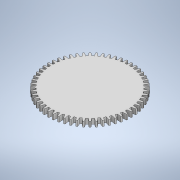
# Autodesk Inventor part: bánh răng 2
Saved by Autodesk Inventor 2020 (Build 240168000, 168)
## iProperties
Created: 2022-11-27
Part Number: bánh răng 2
Material: Generic
Document SubType Name: Modeling
Designer: ADMIN
Density: 1 g/cm^3
Appearance: Default
Author: ADMIN
Autodesk Inventor part; units mm, degrees
ref_plane "YZ Plane" through (0, 0, 0) normal (1, 0, 0) x (0, 1, 0)
ref_plane "XZ Plane" through (0, 0, 0) normal (0, 1, 0) x (-1, 0, 0)
ref_plane "XY Plane" through (0, 0, 0) normal (0, 0, 1) x (1, 0, 0)
sketch "Sketch1" plane through (0, 0, 0) normal (0, 1, 0) x (-1, 0, 0)
  arc A0 (32.9962, -0.5) -> (32.9962, 0.5) centre (0, 0) ccw
  line L0 (29.9833, 1) -> (32.9962, 0.5)
  line L1 (29.9833, -1) -> (32.9962, -0.5)
  line L2 (29.6828, -4.3508) -> (32.7328, -4.1913)
  line L3 (29.9068, -2.3634) -> (32.8447, -3.1975)
  arc A1 (32.7328, -4.1913) -> (32.8447, -3.1975) centre (0, 0) ccw
  line L4 (29.0091, -7.6468) -> (32.0577, -7.8298)
  line L5 (29.4541, -5.697) -> (32.2802, -6.8549)
  arc A2 (32.0577, -7.8298) -> (32.2802, -6.8549) centre (0, 0) ccw
  line L6 (27.9705, -10.8467) -> (30.9794, -11.3699)
  line L7 (28.631, -8.959) -> (31.3097, -10.426)
  arc A3 (30.9794, -11.3699) -> (31.3097, -10.426) centre (0, 0) ccw
  line L8 (26.5802, -13.9102) -> (29.5116, -14.767)
  line L9 (27.4479, -12.1083) -> (29.9455, -13.866)
  arc A4 (29.5116, -14.767) -> (29.9455, -13.866) centre (0, 0) ccw
  line L10 (24.8556, -16.7988) -> (27.6727, -17.9784)
  line L11 (25.9196, -15.1054) -> (28.2047, -17.1317)
  arc A5 (27.6727, -17.9784) -> (28.2047, -17.1317) centre (0, 0) ccw
  line L12 (22.8184, -19.4761) -> (25.4857, -20.9637)
  line L13 (24.0654, -17.9125) -> (26.1092, -20.1819)
  arc A6 (25.4857, -20.9637) -> (26.1092, -20.1819) centre (0, 0) ccw
  line L14 (20.4943, -21.9085) -> (22.9783, -23.6854)
  line L15 (21.9085, -20.4943) -> (23.6854, -22.9783)
  arc A7 (22.9783, -23.6854) -> (23.6854, -22.9783) centre (0, 0) ccw
  line L16 (17.9125, -24.0654) -> (20.1819, -26.1092)
  line L17 (19.4761, -22.8184) -> (20.9637, -25.4857)
  arc A8 (20.1819, -26.1092) -> (20.9637, -25.4857) centre (0, 0) ccw
  line L18 (15.1054, -25.9196) -> (17.1317, -28.2047)
  line L19 (16.7988, -24.8556) -> (17.9784, -27.6727)
  arc A9 (17.1317, -28.2047) -> (17.9784, -27.6727) centre (0, 0) ccw
  line L20 (12.1083, -27.4479) -> (13.866, -29.9455)
  line L21 (13.9102, -26.5802) -> (14.767, -29.5116)
  arc A10 (13.866, -29.9455) -> (14.767, -29.5116) centre (0, 0) ccw
  line L22 (8.959, -28.631) -> (10.426, -31.3097)
  line L23 (10.8467, -27.9705) -> (11.3699, -30.9794)
  arc A11 (10.426, -31.3097) -> (11.3699, -30.9794) centre (0, 0) ccw
  line L24 (5.697, -29.4541) -> (6.8549, -32.2802)
  line L25 (7.6468, -29.0091) -> (7.8298, -32.0577)
  arc A12 (6.8549, -32.2802) -> (7.8298, -32.0577) centre (0, 0) ccw
  line L26 (2.3634, -29.9068) -> (3.1975, -32.8447)
  line L27 (4.3508, -29.6828) -> (4.1913, -32.7328)
  arc A13 (3.1975, -32.8447) -> (4.1913, -32.7328) centre (0, 0) ccw
  line L28 (-1, -29.9833) -> (-0.5, -32.9962)
  line L29 (1, -29.9833) -> (0.5, -32.9962)
  arc A14 (-0.5, -32.9962) -> (0.5, -32.9962) centre (0, 0) ccw
  line L30 (-4.3508, -29.6828) -> (-4.1913, -32.7328)
  line L31 (-2.3634, -29.9068) -> (-3.1975, -32.8447)
  arc A15 (-4.1913, -32.7328) -> (-3.1975, -32.8447) centre (0, 0) ccw
  line L32 (-7.6468, -29.0091) -> (-7.8298, -32.0577)
  line L33 (-5.697, -29.4541) -> (-6.8549, -32.2802)
  arc A16 (-7.8298, -32.0577) -> (-6.8549, -32.2802) centre (0, 0) ccw
  line L34 (-10.8467, -27.9705) -> (-11.3699, -30.9794)
  line L35 (-8.959, -28.631) -> (-10.426, -31.3097)
  arc A17 (-11.3699, -30.9794) -> (-10.426, -31.3097) centre (0, 0) ccw
  line L36 (-13.9102, -26.5802) -> (-14.767, -29.5116)
  line L37 (-12.1083, -27.4479) -> (-13.866, -29.9455)
  arc A18 (-14.767, -29.5116) -> (-13.866, -29.9455) centre (0, 0) ccw
  line L38 (-16.7988, -24.8556) -> (-17.9784, -27.6727)
  line L39 (-15.1054, -25.9196) -> (-17.1317, -28.2047)
  arc A19 (-17.9784, -27.6727) -> (-17.1317, -28.2047) centre (0, 0) ccw
  line L40 (-19.4761, -22.8184) -> (-20.9637, -25.4857)
  line L41 (-17.9125, -24.0654) -> (-20.1819, -26.1092)
  arc A20 (-20.9637, -25.4857) -> (-20.1819, -26.1092) centre (0, 0) ccw
  line L42 (-21.9085, -20.4943) -> (-23.6854, -22.9783)
  line L43 (-20.4943, -21.9085) -> (-22.9783, -23.6854)
  arc A21 (-23.6854, -22.9783) -> (-22.9783, -23.6854) centre (0, 0) ccw
  line L44 (-24.0654, -17.9125) -> (-26.1092, -20.1819)
  line L45 (-22.8184, -19.4761) -> (-25.4857, -20.9637)
  arc A22 (-26.1092, -20.1819) -> (-25.4857, -20.9637) centre (0, 0) ccw
  line L46 (-25.9196, -15.1054) -> (-28.2047, -17.1317)
  line L47 (-24.8556, -16.7988) -> (-27.6727, -17.9784)
  arc A23 (-28.2047, -17.1317) -> (-27.6727, -17.9784) centre (0, 0) ccw
  line L48 (-27.4479, -12.1083) -> (-29.9455, -13.866)
  line L49 (-26.5802, -13.9102) -> (-29.5116, -14.767)
  arc A24 (-29.9455, -13.866) -> (-29.5116, -14.767) centre (0, 0) ccw
  line L50 (-28.631, -8.959) -> (-31.3097, -10.426)
  line L51 (-27.9705, -10.8467) -> (-30.9794, -11.3699)
  arc A25 (-31.3097, -10.426) -> (-30.9794, -11.3699) centre (0, 0) ccw
  line L52 (-29.4541, -5.697) -> (-32.2802, -6.8549)
  line L53 (-29.0091, -7.6468) -> (-32.0577, -7.8298)
  arc A26 (-32.2802, -6.8549) -> (-32.0577, -7.8298) centre (0, 0) ccw
  line L54 (-29.9068, -2.3634) -> (-32.8447, -3.1975)
  line L55 (-29.6828, -4.3508) -> (-32.7328, -4.1913)
  arc A27 (-32.8447, -3.1975) -> (-32.7328, -4.1913) centre (0, 0) ccw
  line L56 (-29.9833, 1) -> (-32.9962, 0.5)
  line L57 (-29.9833, -1) -> (-32.9962, -0.5)
  arc A28 (-32.9962, 0.5) -> (-32.9962, -0.5) centre (0, 0) ccw
  line L58 (-29.6828, 4.3508) -> (-32.7328, 4.1913)
  line L59 (-29.9068, 2.3634) -> (-32.8447, 3.1975)
  arc A29 (-32.7328, 4.1913) -> (-32.8447, 3.1975) centre (0, 0) ccw
  line L60 (-29.0091, 7.6468) -> (-32.0577, 7.8298)
  line L61 (-29.4541, 5.697) -> (-32.2802, 6.8549)
  arc A30 (-32.0577, 7.8298) -> (-32.2802, 6.8549) centre (0, 0) ccw
  line L62 (-27.9705, 10.8467) -> (-30.9794, 11.3699)
  line L63 (-28.631, 8.959) -> (-31.3097, 10.426)
  arc A31 (-30.9794, 11.3699) -> (-31.3097, 10.426) centre (0, 0) ccw
  line L64 (-26.5802, 13.9102) -> (-29.5116, 14.767)
  line L65 (-27.4479, 12.1083) -> (-29.9455, 13.866)
  arc A32 (-29.5116, 14.767) -> (-29.9455, 13.866) centre (0, 0) ccw
  line L66 (-24.8556, 16.7988) -> (-27.6727, 17.9784)
  line L67 (-25.9196, 15.1054) -> (-28.2047, 17.1317)
  arc A33 (-27.6727, 17.9784) -> (-28.2047, 17.1317) centre (0, 0) ccw
  line L68 (-22.8184, 19.4761) -> (-25.4857, 20.9637)
  line L69 (-24.0654, 17.9125) -> (-26.1092, 20.1819)
  arc A34 (-25.4857, 20.9637) -> (-26.1092, 20.1819) centre (0, 0) ccw
  line L70 (-20.4943, 21.9085) -> (-22.9783, 23.6854)
  line L71 (-21.9085, 20.4943) -> (-23.6854, 22.9783)
  arc A35 (-22.9783, 23.6854) -> (-23.6854, 22.9783) centre (0, 0) ccw
  line L72 (-17.9125, 24.0654) -> (-20.1819, 26.1092)
  line L73 (-19.4761, 22.8184) -> (-20.9637, 25.4857)
  arc A36 (-20.1819, 26.1092) -> (-20.9637, 25.4857) centre (0, 0) ccw
  line L74 (-15.1054, 25.9196) -> (-17.1317, 28.2047)
  line L75 (-16.7988, 24.8556) -> (-17.9784, 27.6727)
  arc A37 (-17.1317, 28.2047) -> (-17.9784, 27.6727) centre (0, 0) ccw
  line L76 (-12.1083, 27.4479) -> (-13.866, 29.9455)
  line L77 (-13.9102, 26.5802) -> (-14.767, 29.5116)
  arc A38 (-13.866, 29.9455) -> (-14.767, 29.5116) centre (0, 0) ccw
  line L78 (-8.959, 28.631) -> (-10.426, 31.3097)
  line L79 (-10.8467, 27.9705) -> (-11.3699, 30.9794)
  arc A39 (-10.426, 31.3097) -> (-11.3699, 30.9794) centre (0, 0) ccw
  line L80 (-5.697, 29.4541) -> (-6.8549, 32.2802)
  line L81 (-7.6468, 29.0091) -> (-7.8298, 32.0577)
  arc A40 (-6.8549, 32.2802) -> (-7.8298, 32.0577) centre (0, 0) ccw
  line L82 (-2.3634, 29.9068) -> (-3.1975, 32.8447)
  line L83 (-4.3508, 29.6828) -> (-4.1913, 32.7328)
  arc A41 (-3.1975, 32.8447) -> (-4.1913, 32.7328) centre (0, 0) ccw
  line L84 (1, 29.9833) -> (0.5, 32.9962)
  line L85 (-1, 29.9833) -> (-0.5, 32.9962)
  arc A42 (0.5, 32.9962) -> (-0.5, 32.9962) centre (0, 0) ccw
  line L86 (4.3508, 29.6828) -> (4.1913, 32.7328)
  line L87 (2.3634, 29.9068) -> (3.1975, 32.8447)
  arc A43 (4.1913, 32.7328) -> (3.1975, 32.8447) centre (0, 0) ccw
  line L88 (7.6468, 29.0091) -> (7.8298, 32.0577)
  line L89 (5.697, 29.4541) -> (6.8549, 32.2802)
  arc A44 (7.8298, 32.0577) -> (6.8549, 32.2802) centre (0, 0) ccw
  line L90 (10.8467, 27.9705) -> (11.3699, 30.9794)
  line L91 (8.959, 28.631) -> (10.426, 31.3097)
  arc A45 (11.3699, 30.9794) -> (10.426, 31.3097) centre (0, 0) ccw
  line L92 (13.9102, 26.5802) -> (14.767, 29.5116)
  line L93 (12.1083, 27.4479) -> (13.866, 29.9455)
  arc A46 (14.767, 29.5116) -> (13.866, 29.9455) centre (0, 0) ccw
  line L94 (16.7988, 24.8556) -> (17.9784, 27.6727)
  line L95 (15.1054, 25.9196) -> (17.1317, 28.2047)
  arc A47 (17.9784, 27.6727) -> (17.1317, 28.2047) centre (0, 0) ccw
  line L96 (19.4761, 22.8184) -> (20.9637, 25.4857)
  line L97 (17.9125, 24.0654) -> (20.1819, 26.1092)
  arc A48 (20.9637, 25.4857) -> (20.1819, 26.1092) centre (0, 0) ccw
  line L98 (21.9085, 20.4943) -> (23.6854, 22.9783)
  line L99 (20.4943, 21.9085) -> (22.9783, 23.6854)
  arc A49 (23.6854, 22.9783) -> (22.9783, 23.6854) centre (0, 0) ccw
  line L100 (24.0654, 17.9125) -> (26.1092, 20.1819)
  line L101 (22.8184, 19.4761) -> (25.4857, 20.9637)
  arc A50 (26.1092, 20.1819) -> (25.4857, 20.9637) centre (0, 0) ccw
  line L102 (25.9196, 15.1054) -> (28.2047, 17.1317)
  line L103 (24.8556, 16.7988) -> (27.6727, 17.9784)
  arc A51 (28.2047, 17.1317) -> (27.6727, 17.9784) centre (0, 0) ccw
  line L104 (27.4479, 12.1083) -> (29.9455, 13.866)
  line L105 (26.5802, 13.9102) -> (29.5116, 14.767)
  arc A52 (29.9455, 13.866) -> (29.5116, 14.767) centre (0, 0) ccw
  line L106 (28.631, 8.959) -> (31.3097, 10.426)
  line L107 (27.9705, 10.8467) -> (30.9794, 11.3699)
  arc A53 (31.3097, 10.426) -> (30.9794, 11.3699) centre (0, 0) ccw
  line L108 (29.4541, 5.697) -> (32.2802, 6.8549)
  line L109 (29.0091, 7.6468) -> (32.0577, 7.8298)
  arc A54 (32.2802, 6.8549) -> (32.0577, 7.8298) centre (0, 0) ccw
  line L110 (29.9068, 2.3634) -> (32.8447, 3.1975)
  line L111 (29.6828, 4.3508) -> (32.7328, 4.1913)
  arc A55 (32.8447, 3.1975) -> (32.7328, 4.1913) centre (0, 0) ccw
  arc A56 (22.8184, 19.4761) -> (21.9085, 20.4943) centre (0, 0) ccw
  arc A57 (20.4943, 21.9085) -> (19.4761, 22.8184) centre (0, 0) ccw
  arc A58 (17.9125, 24.0654) -> (16.7988, 24.8556) centre (0, 0) ccw
  arc A59 (15.1054, 25.9196) -> (13.9102, 26.5802) centre (0, 0) ccw
  arc A60 (12.1083, 27.4479) -> (10.8467, 27.9705) centre (0, 0) ccw
  arc A61 (8.959, 28.631) -> (7.6468, 29.0091) centre (0, 0) ccw
  arc A62 (5.697, 29.4541) -> (4.3508, 29.6828) centre (0, 0) ccw
  arc A63 (2.3634, 29.9068) -> (1, 29.9833) centre (0, 0) ccw
  arc A64 (-1, 29.9833) -> (-2.3634, 29.9068) centre (0, 0) ccw
  arc A65 (-4.3508, 29.6828) -> (-5.697, 29.4541) centre (0, 0) ccw
  arc A66 (-7.6468, 29.0091) -> (-8.959, 28.631) centre (0, 0) ccw
  arc A67 (-10.8467, 27.9705) -> (-12.1083, 27.4479) centre (0, 0) ccw
  arc A68 (-13.9102, 26.5802) -> (-15.1054, 25.9196) centre (0, 0) ccw
  arc A69 (-16.7988, 24.8556) -> (-17.9125, 24.0654) centre (0, 0) ccw
  arc A70 (-19.4761, 22.8184) -> (-20.4943, 21.9085) centre (0, 0) ccw
  arc A71 (-21.9085, 20.4943) -> (-22.8184, 19.4761) centre (0, 0) ccw
  arc A72 (-24.0654, 17.9125) -> (-24.8556, 16.7988) centre (0, 0) ccw
  arc A73 (-25.9196, 15.1054) -> (-26.5802, 13.9102) centre (0, 0) ccw
  arc A74 (-27.4479, 12.1083) -> (-27.9705, 10.8467) centre (0, 0) ccw
  arc A75 (-28.631, 8.959) -> (-29.0091, 7.6468) centre (0, 0) ccw
  arc A76 (-29.4541, 5.697) -> (-29.6828, 4.3508) centre (0, 0) ccw
  arc A77 (-29.9068, 2.3634) -> (-29.9833, 1) centre (0, 0) ccw
  arc A78 (-29.9833, -1) -> (-29.9068, -2.3634) centre (0, 0) ccw
  arc A79 (-29.6828, -4.3508) -> (-29.4541, -5.697) centre (0, 0) ccw
  arc A80 (-29.0091, -7.6468) -> (-28.631, -8.959) centre (0, 0) ccw
  arc A81 (-27.9705, -10.8467) -> (-27.4479, -12.1083) centre (0, 0) ccw
  arc A82 (-26.5802, -13.9102) -> (-25.9196, -15.1054) centre (0, 0) ccw
  arc A83 (-24.8556, -16.7988) -> (-24.0654, -17.9125) centre (0, 0) ccw
  arc A84 (-22.8184, -19.4761) -> (-21.9085, -20.4943) centre (0, 0) ccw
  arc A85 (-20.4943, -21.9085) -> (-19.4761, -22.8184) centre (0, 0) ccw
  arc A86 (-17.9125, -24.0654) -> (-16.7988, -24.8556) centre (0, 0) ccw
  arc A87 (-15.1054, -25.9196) -> (-13.9102, -26.5802) centre (0, 0) ccw
  arc A88 (-12.1083, -27.4479) -> (-10.8467, -27.9705) centre (0, 0) ccw
  arc A89 (-8.959, -28.631) -> (-7.6468, -29.0091) centre (0, 0) ccw
  arc A90 (-5.697, -29.4541) -> (-4.3508, -29.6828) centre (0, 0) ccw
  arc A91 (-2.3634, -29.9068) -> (-1, -29.9833) centre (0, 0) ccw
  arc A92 (1, -29.9833) -> (2.3634, -29.9068) centre (0, 0) ccw
  arc A93 (4.3508, -29.6828) -> (5.697, -29.4541) centre (0, 0) ccw
  arc A94 (7.6468, -29.0091) -> (8.959, -28.631) centre (0, 0) ccw
  arc A95 (10.8467, -27.9705) -> (12.1083, -27.4479) centre (0, 0) ccw
  arc A96 (13.9102, -26.5802) -> (15.1054, -25.9196) centre (0, 0) ccw
  arc A97 (16.7988, -24.8556) -> (17.9125, -24.0654) centre (0, 0) ccw
  arc A98 (19.4761, -22.8184) -> (20.4943, -21.9085) centre (0, 0) ccw
  arc A99 (21.9085, -20.4943) -> (22.8184, -19.4761) centre (0, 0) ccw
  arc A100 (24.0654, -17.9125) -> (24.8556, -16.7988) centre (0, 0) ccw
  arc A101 (25.9196, -15.1054) -> (26.5802, -13.9102) centre (0, 0) ccw
  arc A102 (27.4479, -12.1083) -> (27.9705, -10.8467) centre (0, 0) ccw
  arc A103 (28.631, -8.959) -> (29.0091, -7.6468) centre (0, 0) ccw
  arc A104 (29.4541, -5.697) -> (29.6828, -4.3508) centre (0, 0) ccw
  arc A105 (24.8556, 16.7988) -> (24.0654, 17.9125) centre (0, 0) ccw
  arc A106 (26.5802, 13.9102) -> (25.9196, 15.1054) centre (0, 0) ccw
  arc A107 (27.9705, 10.8467) -> (27.4479, 12.1083) centre (0, 0) ccw
  arc A108 (29.0091, 7.6468) -> (28.631, 8.959) centre (0, 0) ccw
  arc A109 (29.6828, 4.3508) -> (29.4541, 5.697) centre (0, 0) ccw
  arc A110 (29.9068, -2.3634) -> (29.9833, -1) centre (0, 0) ccw
  arc A111 (29.9833, 1) -> (29.9068, 2.3634) centre (0, 0) ccw
  dimension "d0" = 66
  dimension "d11" = 360
  constraints: 224 end point, 112 equal length, 112 point on circle, 57 coincident, 56 centre point, 56 concentric, 393 other
  measures "d0" diameter of A0
extrude "Extrusion2" add sketch "Sketch1" along normal blind 4
body "Solid2"
